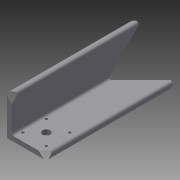
# Autodesk Inventor part: L beam concept
Saved by Autodesk Inventor 2015 (Build 190159000, 159)
## iProperties
Created: 2015-02-14
Part Number: L beam concept
Material: Generic
Document SubType Name: Modeling
Designer: chapale16
Density: 1 g/cm^3
Appearance: Default
Author: chapale16
Autodesk Inventor part; units mm, degrees
ref_plane "YZ Plane" through (0, 0, 0) normal (1, 0, 0) x (0, 1, 0)
ref_plane "XZ Plane" through (0, 0, 0) normal (0, 1, 0) x (-1, 0, 0)
ref_plane "XY Plane" through (0, 0, 0) normal (0, 0, 1) x (1, 0, 0)
sketch "Sketch1" plane through (0, 0, 0) normal (0, 0, 1) x (1, 0, 0)
  line L0 (0, 0) -> (0, 50.8)
  line L1 (0, 0) -> (50.8, 0)
  line L2 (0, 50.8) -> (6.35, 50.8)
  line L3 (6.35, 50.8) -> (6.35, 0)
  line L4 (6.35, 0) -> (0, 0)
  line L5 (0, 0) -> (0, 50.8)
  line L6 (0, 0) -> (50.8, 0)
  line L7 (50.8, 0) -> (50.8, 6.35)
  line L8 (50.8, 6.35) -> (0, 6.35)
  line L9 (0, 6.35) -> (0, 0)
  dimension "d0" = 50.8
  dimension "d1" = 50.8
  dimension "d2" = 6.35
  dimension "d3" = 6.35
  constraints: 20 end point, 4 parallel, 3 horizontal, 2 perpendicular, 1 point on line, 1 vertical
  measures "d0" distance of L0.start L0.end
  measures "d1" distance of L0.start L1.end
  measures "d2" distance of L3.end L4.end
  measures "d3" distance of L7.end L6.end
extrude "Extrusion1" add sketch "Sketch1" along normal blind 101.6
fillet "Fillet1" radius 3.175 1 edges at (6.35, 50.8, 50.8)
fillet "Fillet2" radius 3.175 1 edges at (50.8, 6.35, 50.8)
fillet "Fillet3" radius 3.175 1 edges at (6.35, 6.35, 50.8)
sketch "Sketch2" plane through (47.625, 6.35, 101.6) normal (0, 1, 0) x (1, 0, 0)
  circle A0 centre (-21.7932, 25.4) radius 5.0038 projected
  line L0 (-47.625, 50.8) -> (-47.625, 101.6) projected
  line L1 (-47.625, 101.6) -> (-73.025, 101.6) projected
  line L2 (-73.025, 101.6) -> (-73.025, 0) projected
  line L3 (-73.025, 0) -> (3.6068, 0) projected
  line L4 (3.6068, 0) -> (3.6068, 50.8) projected
  line L5 (3.6068, 50.8) -> (-45.308, 50.8) projected
  line L6 (-45.308, 101.6) -> (-45.308, 50.8) projected
  line L7 (-45.4152, 101.6) -> (-45.308, 101.6) projected
  line L8 (-45.4152, 50.8) -> (-45.4152, 101.6) projected
  line L9 (-45.4152, 50.8) -> (-47.5178, 50.8) projected
  line L10 (-47.5178, 50.8) -> (-47.625, 50.8) projected
  circle A1 centre (-6.5659, 40.6273) radius 1.651 projected
  circle A2 centre (-6.5659, 10.1727) radius 1.651 projected
  circle A3 centre (-37.0205, 10.1727) radius 1.651 projected
  circle A4 centre (-37.0205, 40.6273) radius 1.651 projected
  line L11 (-38.1, 0) -> (-38.1, 101.6) projected
  line L12 (0, 0) -> (-38.1, 0) projected
  line L13 (0, 101.6) -> (0, 0) projected
  line L14 (0, 101.6) -> (-38.1, 101.6) projected
extrude "Extrusion2" cut sketch "Sketch2" along normal mid plane 25.4 contours A0 | L11 A3 | A3 L11 | L11 A4 | A4 L11 | A1 | A2
sketch "Sketch3" plane through (0, 0, 0) normal (0, 0, -1) x (-1, 0, 0)
  arc A0 (-47.625, 6.35) -> (-50.8, 3.175) centre (-47.625, 3.175) ccw projected
  line L0 (-50.8, 0) -> (-50.8, 3.175) projected
  line L1 (0, 0) -> (-50.8, 0) projected
  line L2 (0, 50.8) -> (0, 0) projected
  line L3 (-3.175, 50.8) -> (0, 50.8) projected
  arc A1 (-3.175, 50.8) -> (-6.35, 47.625) centre (-3.175, 47.625) ccw projected
  line L4 (-6.35, 9.525) -> (-6.35, 47.625) projected
  arc A2 (-9.525, 6.35) -> (-6.35, 9.525) centre (-9.525, 9.525) ccw projected
  line L5 (-47.625, 6.35) -> (-9.525, 6.35) projected
extrude "Extrusion3" add sketch "Sketch3" along normal blind 63.5
body "Solid1"
